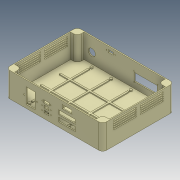
# Autodesk Inventor part: caixa-gabinete-fundo
Saved by Autodesk Inventor 2017 (Build 210142000, 142)
## iProperties
Created: 2018-08-05
Part Number: caixa-gabinete-fundo
Material: ABS Plastic
Document SubType Name: Modeling
Designer: Luiz Gustavo
Density: 1.06 g/cm^3
Appearance: Smooth - Ash
Author: Luiz Gustavo
Autodesk Inventor part; units mm, degrees
ref_plane "YZ Plane" through (0, 0, 0) normal (1, 0, 0) x (0, 1, 0)
ref_plane "XZ Plane" through (0, 0, 0) normal (0, 1, 0) x (-1, 0, 0)
sketch "Sketch1" plane through (0, 0, 0) normal (0, 0, 1) x (1, 0, 0)
  line L0 (-152.5, -112.5) -> (152.5, -112.5)
  line L1 (152.5, -112.5) -> (152.5, 112.5)
  line L2 (152.5, 112.5) -> (-152.5, 112.5)
  line L3 (-152.5, 112.5) -> (-152.5, -112.5)
  line L4 (-152.5, -112.5) -> (152.5, 112.5) construction
  line L5 (152.5, -112.5) -> (-152.5, 112.5) construction
  point P0 (0, 0)
  dimension "d4" = 305
  dimension "d5" = 225
  constraints: 12 end point, 2 midpoint, 2 parallel, 1 horizontal, 1 perpendicular
  measures "d4" distance of L2.end L1.end
  measures "d5" distance of L1.end L0.end
extrude "Extrusion1" add sketch "Sketch1" along normal blind 78
fillet "Fillet1" radius 12 4 edges at (-152.5, -112.5, 39) (152.5, -112.5, 39) (152.5, 112.5, 39) (-152.5, 112.5, 39)
sketch "Sketch2" plane through (0, 0, 78) normal (0, 0, 1) x (1, 0, 0)
  arc A0 (-140.5, 112.5) -> (-152.5, 100.5) centre (-140.5, 100.5) ccw construction
  line L0 (-152.5, 100.5) -> (-152.5, -100.5) construction
  arc A1 (-152.5, -100.5) -> (-140.5, -112.5) centre (-140.5, -100.5) ccw construction
  line L1 (-140.5, -112.5) -> (140.5, -112.5) construction
  arc A2 (140.5, -112.5) -> (152.5, -100.5) centre (140.5, -100.5) ccw construction
  line L2 (152.5, -100.5) -> (152.5, 100.5) construction
  arc A3 (152.5, 100.5) -> (140.5, 112.5) centre (140.5, 100.5) ccw construction
  line L3 (140.5, 112.5) -> (-140.5, 112.5) construction
  circle A4 centre (-140.5, -100.5) radius 12
  circle A5 centre (-140.5, 100.5) radius 12
  arc A6 (-140.5, 112.5) -> (-152.5, 100.5) centre (-140.5, 100.5) ccw projected
  circle A7 centre (140.5, 100.5) radius 12
  line L4 (152.5, -100.5) -> (152.5, 100.5) construction
  circle A8 centre (140.5, -100.5) radius 12
  line L5 (-149.5, 109.5) -> (-128.5, 109.5) construction
  line L6 (149.5, 109.5) -> (149.5, 88.5) construction
  line L7 (149.5, -109.5) -> (128.5, -109.5) construction
  line L8 (-149.5, -109.5) -> (-149.5, -88.5) construction
  line L9 (-149.5, 109.5) -> (149.5, -109.5) construction
  line L10 (149.5, 109.5) -> (-149.5, -109.5) construction
  line L11 (-140.5, -88.5) -> (-149.5, -88.5)
  line L12 (-128.5, -100.5) -> (-128.5, -109.5)
  line L13 (-140.5, 88.5) -> (-149.5, 88.5)
  line L14 (-128.5, 109.5) -> (-128.5, 100.5)
  line L15 (128.5, 109.5) -> (128.5, 100.5)
  line L16 (149.5, 88.5) -> (140.5, 88.5)
  line L17 (140.5, -88.5) -> (149.5, -88.5)
  line L18 (128.5, -100.5) -> (128.5, -109.5)
  line L19 (128.5, -109.5) -> (-128.5, -109.5)
  line L20 (149.5, -88.5) -> (149.5, -109.5) construction
  line L21 (149.5, 88.5) -> (149.5, -88.5)
  line L22 (128.5, 109.5) -> (149.5, 109.5) construction
  line L23 (-128.5, 109.5) -> (128.5, 109.5)
  line L24 (-149.5, 88.5) -> (-149.5, 109.5) construction
  line L25 (-149.5, -88.5) -> (-149.5, 88.5)
  line L26 (-128.5, -109.5) -> (-149.5, -109.5) construction
  point P0 (0, 0)
  dimension "d11" = 3
  dimension "d12" = 3
  constraints: 44 end point, 33 perpendicular, 18 parallel, 9 point on circle, 9 tangent, 4 centre point, 4 coincident, 3 horizontal, 2 concentric, 2 midpoint, 1 point on line
  measures "d11" distance between parallel lines of L1 L7
  measures "d12" distance between parallel lines of L2 L6
extrude "Extrusion2" cut sketch "Sketch2" against normal blind 75 contours A4 L11 L25 L13 A5 L14 L23 L15 A7 L16 L21 L17 A8 L18 L19 L12
ref_plane "Work Plane1" through (0, 0, -1) normal (0, 0, 1) x (1, 0, 0)
sketch "Sketch4" plane through (0, 0, -1) normal (0, 0, 1) x (1, 0, 0)
  line L0 (-95.5, -90) -> (-90.5, -90)
  line L1 (-90.5, -90) -> (-90.5, 90)
  line L2 (-90.5, 90) -> (-95.5, 90)
  line L3 (-95.5, 90) -> (-95.5, -90)
  line L4 (0, 0) -> (-95.5, 0) construction
  line L5 (-33.5, -90) -> (-28.5, -90)
  line L6 (-28.5, -90) -> (-28.5, 90)
  line L7 (-28.5, 90) -> (-33.5, 90)
  line L8 (-33.5, 90) -> (-33.5, -90)
  line L9 (28.5, -90) -> (33.5, -90)
  line L10 (33.5, -90) -> (33.5, 90)
  line L11 (33.5, 90) -> (28.5, 90)
  line L12 (28.5, 90) -> (28.5, -90)
  line L13 (90.5, -90) -> (95.5, -90)
  line L14 (95.5, -90) -> (95.5, 90)
  line L15 (95.5, 90) -> (90.5, 90)
  line L16 (90.5, 90) -> (90.5, -90)
  line L17 (0, 0) -> (0, 90) construction
  line L18 (0, 90) -> (28.5, 90) construction
  line L19 (125, 32.5) -> (-125, 32.5)
  line L20 (-125, 32.5) -> (-125, 27.5)
  line L21 (-125, 27.5) -> (125, 27.5)
  line L22 (125, 27.5) -> (125, 32.5)
  line L23 (-125, 30) -> (125, 30) construction
  line L24 (125, -32.5) -> (-125, -32.5)
  line L25 (-125, -32.5) -> (-125, -27.5)
  line L26 (-125, -27.5) -> (125, -27.5)
  line L27 (125, -27.5) -> (125, -32.5)
  circle A0 centre (-93, -98) radius 4
  line L28 (-93, -98) -> (-93, -90) construction
  line L29 (-93, 90) -> (-93, 98) construction
  circle A1 centre (-93, 98) radius 4
  circle A2 centre (-31, -98) radius 4
  circle A3 centre (-31, 98) radius 4
  circle A4 centre (31, -98) radius 4
  circle A5 centre (31, 98) radius 4
  circle A6 centre (93, -98) radius 4
  circle A7 centre (93, 98) radius 4
  point P0 (-33.5, 0)
  point P1 (28.5, 0)
  point P2 (90.5, 0)
  point P3 (0, 32.5)
  dimension "d16" = 5
  dimension "d17" = 180
  dimension "d20" = 62
  dimension "d25" = 5
  dimension "d26" = 60
  dimension "d27" = 250
  dimension "d28" = 8
  dimension "d29" = 8
  dimension "d32" = 62
  constraints: 60 end point, 8 centre point, 6 midpoint, 5 horizontal, 4 parallel, 4 symmetric about line, 3 perpendicular, 3 vertical, 1 coincident, 1 collinear, 1 equal radius, 1 point on line, 40 other
  measures "d16" distance between parallel lines of L1 L3
  measures "d17" distance between parallel lines of L0 L2
  measures "d20" distance of L0.start L5.start
  measures "d25" distance of L19.end L20.end
  measures "d26" distance between parallel lines of L2 L23
  measures "d27" distance of L19.start L19.end
  measures "d28" diameter of A0
  measures "d29" distance from line of L0 L28.start
  measures "d32" distance of L28.start A2.centre
extrude "Extrusion3" add sketch "Sketch4" along normal blind 7 contours L3 L24 L1 L0 | L24 L25 L26 L3 | L3 L26 L1 L24 | L1 L26 L8 L24 | L3 L21 L1 L26 | L24 L6 L5 L8 | L8 L26 L6 L24 | L21 L20 L19 L3 | L3 L19 L1 L21 | L1 L19 L8 L21 | L8 L21 L6 L26 | L6 L26 L12 L24 | L3 L2 L1 L19 | L8 L19 L6 L21 | L24 L10 L9 L12 | L12 L26 L10 L24 | L8 L7 L6 L19 | L6 L19 L12 L21 | L12 L21 L10 L26 | L10 L26 L16 L24 | L12 L19 L10 L21 | L24 L14 L13 L16 | L16 L26 L14 L24 | L12 L11 L10 L19 | L10 L19 L16 L21 | L16 L21 L14 L26 | L14 L26 L27 L24 | L16 L19 L14 L21 | L16 L15 L14 L19 | L14 L19 L22 L21 | A0 | A1 | A2 | A3 | A4 | A5 | A6 | A7
sketch "Sketch5" plane through (-140.5, 112.5, 0) normal (0, 1, 0) x (1, 0, 0)
  line L0 (243, -22.5) -> (171, -22.5)
  line L1 (171, -22.5) -> (171, -47.5)
  line L2 (171, -47.5) -> (243, -47.5)
  line L3 (243, -47.5) -> (243, -22.5)
  line L4 (243, -22.5) -> (171, -47.5) construction
  line L5 (171, -22.5) -> (243, -47.5) construction
  line L6 (244.5, -19.5) -> (169.5, -19.5) construction
  line L7 (169.5, -19.5) -> (169.5, -50.5) construction
  line L8 (169.5, -50.5) -> (244.5, -50.5) construction
  line L9 (244.5, -50.5) -> (244.5, -19.5) construction
  line L10 (244.5, -19.5) -> (169.5, -50.5) construction
  line L11 (169.5, -19.5) -> (244.5, -50.5) construction
  circle A0 centre (244.5, -50.5) radius 1.5
  circle A1 centre (169.5, -19.5) radius 1.5
  circle A2 centre (169.5, -50.5) radius 1.5
  circle A3 centre (244.5, -19.5) radius 1.5
  circle A4 centre (37, -35) radius 11
  line L12 (37, -35) -> (207, -35) construction
  line L13 (104.5, -61.25) -> (89.5, -61.25)
  line L14 (89.5, -61.25) -> (89.5, -68.75)
  line L15 (89.5, -68.75) -> (104.5, -68.75)
  line L16 (104.5, -68.75) -> (104.5, -61.25)
  line L17 (12, -78) -> (12, -3) construction
  circle A5 centre (111, -65) radius 1.5
  circle A6 centre (83, -65) radius 1.5
  line L18 (111, -65) -> (83, -65) construction
  line L19 (97, -68.75) -> (97, -61.25) construction
  point P0 (140.5, 0)
  point P1 (104.5, -65)
  dimension "d39" = 75
  dimension "d40" = 31
  dimension "d41" = 25
  dimension "d42" = 72
  dimension "d43" = 3
  dimension "d44" = 22
  dimension "d45" = 15
  dimension "d46" = 7.5
  dimension "d49" = 35
  dimension "d52" = 25
  dimension "d115" = 3
  dimension "d116" = 28
  dimension "d117" = 30
  dimension "d118" = 60
  dimension "d119" = 110
  constraints: 38 end point, 9 midpoint, 7 centre point, 6 parallel, 5 horizontal, 4 coincident, 4 equal radius, 3 perpendicular, 1 point on line, 1 other
  measures "d39" distance of L7.end L8.end
  measures "d40" distance of L6.end L7.end
  measures "d41" distance of L0.end L1.end
  measures "d42" distance of L1.end L2.end
  measures "d43" diameter of A0
  measures "d44" diameter of A4
  measures "d45" distance of L15.end L14.end
  measures "d46" distance of L14.end L13.end
  measures "d49" distance from line of point (140.5, 0) L12
  measures "d52" distance from line of L17 L12.start
  measures "d115" diameter of A5
  measures "d116" distance of L18.start L18.end
  measures "d117" distance between parallel lines of L12 L18
  measures "d118" distance from line of L19 L12.start
  measures "d119" distance from line of L19 point (207, -35)
extrude "Extrusion4" cut sketch "Sketch5" against normal up to surface (3 mm away)
sketch "Sketch6" plane through (0, 0, 0) normal (0, 0, 1) x (1, 0, 0)
  line L0 (128.5, -109.5) -> (-128.5, -109.5) construction
  line L1 (124, -109.5) -> (101, -109.5)
  line L2 (101, -109.5) -> (101, -104.5)
  line L3 (101, -104.5) -> (124, -104.5)
  line L4 (124, -104.5) -> (124, -109.5)
  line L5 (0, -109.5) -> (0, 0) construction
  line L6 (-124, -109.5) -> (-101, -109.5)
  line L7 (-101, -109.5) -> (-101, -104.5)
  line L8 (-101, -104.5) -> (-124, -104.5)
  line L9 (-124, -104.5) -> (-124, -109.5)
  dimension "d55" = 23
  dimension "d56" = 5
  dimension "d57" = 202
  constraints: 18 end point, 4 symmetric about line, 2 parallel, 1 horizontal, 1 midpoint, 1 perpendicular, 1 point on line, 1 vertical
  measures "d55" distance of L2.end L3.end
  measures "d56" distance of L1.end L2.end
  measures "d57" distance between parallel lines of L7 L2
extrude "Extrusion5" add sketch "Sketch6" along normal blind 70
sketch "Sketch7" plane through (-140.5, -112.5, 0) normal (0, -1, 0) x (1, 0, 0)
  line L0 (51.5, 59) -> (79.5, 59)
  line L1 (79.5, 59) -> (79.5, 11)
  line L2 (79.5, 11) -> (51.5, 11)
  line L3 (51.5, 11) -> (51.5, 59)
  line L4 (65.5, 59) -> (65.5, 11) construction
  line L5 (45.5, 35) -> (85.5, 35) construction
  circle A0 centre (45.5, 35) radius 2
  circle A1 centre (85.5, 35) radius 2
  line L6 (85.5, 35) -> (180.5, 35) construction
  line L7 (115.5, 35) -> (115.5, 20) construction
  line L8 (101.5, 20) -> (129.5, 20) construction
  circle A2 centre (101.5, 20) radius 1.5
  circle A3 centre (129.5, 20) radius 1.5
  line L9 (108, 16.25) -> (123, 16.25)
  line L10 (123, 16.25) -> (123, 23.75)
  line L11 (123, 23.75) -> (108, 23.75)
  line L12 (108, 23.75) -> (108, 16.25)
  line L13 (108, 16.25) -> (123, 23.75) construction
  line L14 (123, 16.25) -> (108, 23.75) construction
  circle A4 centre (101.5, 33.5) radius 1.5
  line L15 (123, 37.25) -> (108, 37.25)
  line L16 (108, 37.25) -> (108, 29.75)
  line L17 (108, 29.75) -> (123, 29.75)
  circle A5 centre (129.5, 33.5) radius 1.5
  line L18 (123, 29.75) -> (123, 37.25)
  line L19 (180.5, 56.5) -> (180.5, 14.5) construction
  line L20 (154, 47.5) -> (207, 47.5)
  line L21 (207, 47.5) -> (207, 34.5)
  line L22 (207, 34.5) -> (154, 34.5)
  line L23 (154, 34.5) -> (154, 47.5)
  line L24 (154, 27.5) -> (207, 27.5)
  line L25 (207, 27.5) -> (207, 14.5)
  line L26 (207, 14.5) -> (154, 14.5)
  line L27 (154, 14.5) -> (154, 27.5)
  line L28 (165, 67.5) -> (196, 67.5)
  line L29 (196, 67.5) -> (196, 56.5)
  line L30 (196, 56.5) -> (165, 56.5)
  line L31 (165, 56.5) -> (165, 67.5)
  line L32 (154, 41) -> (207, 41) construction
  line L33 (106.5, 51.25) -> (124.5, 51.25)
  line L34 (124.5, 51.25) -> (124.5, 42.75)
  line L35 (124.5, 42.75) -> (106.5, 42.75)
  line L36 (106.5, 42.75) -> (106.5, 51.25)
  line L37 (106.5, 51.25) -> (124.5, 42.75) construction
  line L38 (124.5, 51.25) -> (106.5, 42.75) construction
  line L39 (115.5, 35) -> (115.5, 47) construction
  line L40 (102.5, 47) -> (128.5, 47) construction
  circle A6 centre (102.5, 47) radius 1.5
  circle A7 centre (128.5, 47) radius 1.5
  point P0 (140.5, 0)
  point P1 (65.5, 35)
  point P2 (180.5, 41)
  dimension "d60" = 28
  dimension "d61" = 48
  dimension "d62" = 40
  dimension "d63" = 4
  dimension "d64" = 28
  dimension "d65" = 3
  dimension "d67" = 7.5
  dimension "d68" = 15
  dimension "d69" = 35
  dimension "d70" = 50
  dimension "d72" = 25
  dimension "d73" = 15
  dimension "d76" = 13.5
  dimension "d85" = 53
  dimension "d86" = 13
  dimension "d87" = 31
  dimension "d88" = 11
  dimension "d89" = 20
  dimension "d90" = 22
  dimension "d91" = 40
  dimension "d92" = 6
  dimension "d110" = 8.5
  dimension "d111" = 18
  dimension "d112" = 26
  dimension "d113" = 12
  dimension "d114" = 3
  constraints: 82 end point, 16 midpoint, 12 parallel, 10 horizontal, 8 centre point, 6 coincident, 6 perpendicular, 4 vertical, 3 equal radius, 3 point on line, 2 equal length, 12 other
  measures "d60" distance of L0.start L0.end
  measures "d61" distance of L0.end L1.end
  measures "d62" distance of L5.start L5.end
  measures "d63" diameter of A0
  measures "d64" distance of L8.start L8.end
  measures "d65" diameter of A2
  measures "d67" distance of L10.end L9.end
  measures "d68" distance of L7.start L7.end
  measures "d69" distance from line of point (140.5, 0) L6
  measures "d70" distance of L7.start point (65.5, 35)
  measures "d72" horizontal distance of point (140.5, 0) L7.end
  measures "d73" distance of L9.start L9.end
  measures "d76" distance of A2.centre A4.centre
  measures "d85" distance of L20.start L20.end
  measures "d86" distance of L20.end L21.end
  measures "d87" distance of L28.start L28.end
  measures "d88" distance of L28.end L29.end
  measures "d89" distance between parallel lines of L22 L26
  measures "d90" distance between parallel lines of L30 L22
  measures "d91" horizontal distance of point (140.5, 0) point (180.5, 41)
  measures "d92" distance between parallel lines of L6 L32
  measures "d110" distance of L33.end L34.end
  measures "d111" distance of L34.end L35.end
  measures "d112" distance of L40.start L40.end
  measures "d113" distance of L39.end L7.start
  measures "d114" diameter of A6
extrude "Extrusion6" cut sketch "Sketch7" against normal up to surface (3 mm away)
sketch "Sketch8" plane through (152.5, -100.5, 0) normal (1, 0, 0) x (0, 0, -1)
  line L0 (-70, 23) -> (-70, 93) construction
  line L1 (-71.5, 23) -> (-71.5, 93)
  line L2 (-68.5, 93) -> (-68.5, 23)
  arc A0 (-71.5, 23) -> (-68.5, 23) centre (-70, 23) ccw
  arc A1 (-68.5, 93) -> (-71.5, 93) centre (-70, 93) ccw
  line L3 (-70, 108) -> (-70, 178) construction
  line L4 (-71.5, 108) -> (-71.5, 178)
  line L5 (-68.5, 178) -> (-68.5, 108)
  arc A2 (-71.5, 108) -> (-68.5, 108) centre (-70, 108) ccw
  arc A3 (-68.5, 178) -> (-71.5, 178) centre (-70, 178) ccw
  line L6 (-70, 93) -> (-70, 108) construction
  line L7 (0, 100.5) -> (-70, 100.5) construction
  line L8 (-64, 108) -> (-64, 178) construction
  line L9 (-65.5, 108) -> (-65.5, 178)
  line L10 (-62.5, 178) -> (-62.5, 108)
  arc A4 (-65.5, 108) -> (-62.5, 108) centre (-64, 108) ccw
  arc A5 (-62.5, 178) -> (-65.5, 178) centre (-64, 178) ccw
  line L11 (-64, 23) -> (-64, 93) construction
  line L12 (-65.5, 23) -> (-65.5, 93)
  line L13 (-62.5, 93) -> (-62.5, 23)
  arc A6 (-65.5, 23) -> (-62.5, 23) centre (-64, 23) ccw
  arc A7 (-62.5, 93) -> (-65.5, 93) centre (-64, 93) ccw
  line L14 (-58, 108) -> (-58, 178) construction
  line L15 (-59.5, 108) -> (-59.5, 178)
  line L16 (-56.5, 178) -> (-56.5, 108)
  arc A8 (-59.5, 108) -> (-56.5, 108) centre (-58, 108) ccw
  arc A9 (-56.5, 178) -> (-59.5, 178) centre (-58, 178) ccw
  line L17 (-58, 23) -> (-58, 93) construction
  line L18 (-59.5, 23) -> (-59.5, 93)
  line L19 (-56.5, 93) -> (-56.5, 23)
  arc A10 (-59.5, 23) -> (-56.5, 23) centre (-58, 23) ccw
  arc A11 (-56.5, 93) -> (-59.5, 93) centre (-58, 93) ccw
  line L20 (-52, 108) -> (-52, 178) construction
  line L21 (-53.5, 108) -> (-53.5, 178)
  line L22 (-50.5, 178) -> (-50.5, 108)
  arc A12 (-53.5, 108) -> (-50.5, 108) centre (-52, 108) ccw
  arc A13 (-50.5, 178) -> (-53.5, 178) centre (-52, 178) ccw
  line L23 (-52, 23) -> (-52, 93) construction
  line L24 (-53.5, 23) -> (-53.5, 93)
  line L25 (-50.5, 93) -> (-50.5, 23)
  arc A14 (-53.5, 23) -> (-50.5, 23) centre (-52, 23) ccw
  arc A15 (-50.5, 93) -> (-53.5, 93) centre (-52, 93) ccw
  line L26 (-46, 108) -> (-46, 178) construction
  line L27 (-47.5, 108) -> (-47.5, 178)
  line L28 (-44.5, 178) -> (-44.5, 108)
  arc A16 (-47.5, 108) -> (-44.5, 108) centre (-46, 108) ccw
  arc A17 (-44.5, 178) -> (-47.5, 178) centre (-46, 178) ccw
  line L29 (-46, 23) -> (-46, 93) construction
  line L30 (-47.5, 23) -> (-47.5, 93)
  line L31 (-44.5, 93) -> (-44.5, 23)
  arc A18 (-47.5, 23) -> (-44.5, 23) centre (-46, 23) ccw
  arc A19 (-44.5, 93) -> (-47.5, 93) centre (-46, 93) ccw
  point P0 (-70, 58)
  point P1 (-70, 143)
  point P2 (-64, 143)
  point P3 (-64, 58)
  point P4 (-58, 143)
  point P5 (-58, 58)
  point P6 (-52, 143)
  point P7 (-52, 58)
  point P8 (-46, 143)
  point P9 (-46, 58)
  dimension "d95" = 70
  dimension "d97" = 3
  dimension "d99" = 15
  dimension "d100" = 70
  dimension "d103" = 6
  constraints: 84 end point, 40 point on circle, 20 centre point, 8 tangent, 3 midpoint, 2 collinear, 2 horizontal, 2 parallel, 2 vertical, 1 equal radius, 96 other
  measures "d95" distance of L0.start L0.end
  measures "d97" distance between parallel lines of L2 L1
  measures "d99" distance of L0.end L3.start
  measures "d100" distance of L7.start L7.end
  measures "d103" distance of L4.start L9.start
extrude "Extrusion7" cut sketch "Sketch8" against normal through all
equation "\"d25\" = d16"
equation "\"d26\" = 0.333333 * d17"
equation "\"d32\" = d20"
body "Solid1"
